Autodesk Inventor part; units mm, degrees
(part 2 of 3)
  spline S34 degree 3 poles (-443.5829, -422.363) (-442.2822, -421.8669) (-439.6808, -420.8747) (-435.8139, -419.2967) (-431.976, -417.6498) (-428.1717, -415.9263) (-424.4077, -414.1171) (-421.6079, -412.712) (-419.7704, -411.7206) (-418.9626, -411.3892) (-418.2875, -411.2153) (-417.7698, -411.1447) (-417.2482, -411.1077) (-416.7264, -411.1464) (-416.21, -411.2266) (-415.7059, -411.3678) (-415.2255, -411.5743) (-414.7643, -411.82) (-414.3345, -412.1194) (-413.8232, -412.5931) (-413.2204, -413.2204) (-412.5931, -413.8232) (-412.1194, -414.3345) (-411.82, -414.7643) (-411.5743, -415.2255) (-411.3678, -415.7059) (-411.2266, -416.21) (-411.1464, -416.7264) (-411.1077, -417.2482) (-411.1447, -417.7698) (-411.2153, -418.2875) (-411.3892, -418.9626) (-411.7206, -419.7704) (-412.712, -421.6079) (-414.1171, -424.4077) (-415.9263, -428.1717) (-417.6498, -431.976) (-419.2967, -435.8139) (-420.8747, -439.6808) (-421.8669, -442.2822) (-422.363, -443.5829) knots 0 0 0 0 0.062504 0.125008 0.187512 0.250016 0.31252 0.375023 0.390648 0.406259 0.414073 0.421883 0.429693 0.437504 0.445316 0.453129 0.460938 0.468749 0.476563 0.484374 0.5 0.515626 0.523437 0.531251 0.539062 0.546871 0.554684 0.562496 0.570307 0.578117 0.585927 0.593741 0.609352 0.624977 0.68748 0.749984 0.812488 0.874992 0.937496 1 1 1 1 projected
  arc A38 (-422.363, -443.5829) -> (-415.0093, -450.4704) centre (0, 0) ccw projected
  spline S35 degree 3 poles (-415.0093, -450.4704) (-413.7438, -449.8903) (-411.2129, -448.73) (-407.4575, -446.9025) (-403.7355, -445.0082) (-400.0521, -443.0396) (-396.4144, -440.988) (-393.7126, -439.4028) (-391.9438, -438.2934) (-391.1594, -437.9098) (-390.4971, -437.6922) (-389.9852, -437.5879) (-389.4671, -437.5168) (-388.9439, -437.5214) (-388.4234, -437.5676) (-387.9111, -437.6755) (-387.4182, -437.8501) (-386.9419, -438.0652) (-386.4935, -438.3358) (-385.9523, -438.775) (-385.3098, -439.3616) (-384.6444, -439.922) (-384.1382, -440.4013) (-383.8114, -440.8106) (-383.5361, -441.2547) (-383.2986, -441.7205) (-383.1247, -442.2144) (-383.0109, -442.7244) (-382.9381, -443.2425) (-382.941, -443.7655) (-382.9776, -444.2867) (-383.1069, -444.9717) (-383.3848, -445.7994) (-384.2539, -447.6979) (-385.4728, -450.5835) (-387.032, -454.4578) (-388.503, -458.3667) (-389.8954, -462.3041) (-391.217, -466.266) (-392.037, -468.9267) (-392.4469, -470.257) knots 0 0 0 0 0.062504 0.125008 0.187512 0.250016 0.31252 0.375023 0.390648 0.406259 0.414073 0.421883 0.429693 0.437504 0.445316 0.453129 0.460938 0.468749 0.476563 0.484374 0.5 0.515626 0.523437 0.531251 0.539062 0.546871 0.554684 0.562496 0.570307 0.578117 0.585927 0.593741 0.609352 0.624977 0.68748 0.749984 0.812488 0.874992 0.937496 1 1 1 1 projected
  arc A39 (-392.4469, -470.257) -> (-384.6585, -476.6488) centre (0, 0) ccw projected
  spline S36 degree 3 poles (-384.6585, -476.6488) (-383.4337, -475.9871) (-380.9841, -474.6639) (-377.3563, -472.5947) (-373.7661, -470.461) (-370.2193, -468.2556) (-366.7237, -465.9706) (-364.1313, -464.2121) (-362.4389, -462.9893) (-361.6812, -462.5553) (-361.0346, -462.2948) (-360.5306, -462.1572) (-360.0182, -462.0524) (-359.4958, -462.0227) (-358.9735, -462.0348) (-358.4552, -462.109) (-357.952, -462.251) (-357.4626, -462.4345) (-356.9975, -462.6752) (-356.4287, -463.0781) (-355.7492, -463.6214) (-355.0485, -464.1371) (-354.5121, -464.5822) (-354.1592, -464.9692) (-353.8554, -465.3944) (-353.588, -465.8437) (-353.3822, -466.3252) (-353.2353, -466.8266) (-353.1288, -467.3389) (-353.0974, -467.8609) (-353.0998, -468.3833) (-353.1841, -469.0753) (-353.4072, -469.9195) (-354.1503, -471.8707) (-355.1779, -474.8299) (-356.4804, -478.7979) (-357.6926, -482.7946) (-358.8244, -486.8147) (-359.8842, -490.8545) (-360.5283, -493.5631) (-360.8504, -494.9174) knots 0 0 0 0 0.062504 0.125008 0.187512 0.250016 0.31252 0.375023 0.390648 0.406259 0.414073 0.421883 0.429693 0.437504 0.445316 0.453129 0.460938 0.468749 0.476563 0.484374 0.5 0.515626 0.523437 0.531251 0.539062 0.546871 0.554684 0.562496 0.570307 0.578117 0.585927 0.593741 0.609352 0.624977 0.68748 0.749984 0.812488 0.874992 0.937496 1 1 1 1 projected
  arc A40 (-360.8504, -494.9174) -> (-352.6606, -500.7861) centre (0, 0) ccw projected
  spline S37 degree 3 poles (-352.6606, -500.7861) (-351.4817, -500.0458) (-349.1239, -498.5651) (-345.6391, -496.2631) (-342.1963, -493.8992) (-338.8013, -491.4666) (-335.4626, -488.9578) (-332.9907, -487.0335) (-331.3819, -485.7026) (-330.6543, -485.22) (-330.0261, -484.9178) (-329.5321, -484.7475) (-329.0277, -484.6094) (-328.5084, -484.5457) (-327.9863, -484.5236) (-327.4643, -484.5637) (-326.9529, -484.6725) (-326.4526, -484.8235) (-325.9727, -485.0333) (-325.3788, -485.3981) (-324.6652, -485.8958) (-323.9323, -486.3646) (-323.368, -486.7737) (-322.9905, -487.1368) (-322.6596, -487.5412) (-322.3633, -487.9721) (-322.1265, -488.439) (-321.9471, -488.9298) (-321.8073, -489.434) (-321.7418, -489.9528) (-321.7101, -490.4743) (-321.7489, -491.1704) (-321.9163, -492.0273) (-322.5302, -494.023) (-323.3621, -497.043) (-324.4023, -501.0877) (-325.3505, -505.1551) (-326.217, -509.2406) (-327.0102, -513.3411) (-327.4758, -516.086) (-327.7086, -517.4585) knots 0 0 0 0 0.062504 0.125008 0.187512 0.250016 0.31252 0.375023 0.390648 0.406259 0.414073 0.421883 0.429693 0.437504 0.445316 0.453129 0.460938 0.468749 0.476563 0.484374 0.5 0.515626 0.523437 0.531251 0.539062 0.546871 0.554684 0.562496 0.570307 0.578117 0.585927 0.593741 0.609352 0.624977 0.68748 0.749984 0.812488 0.874992 0.937496 1 1 1 1 projected
  arc A41 (-327.7086, -517.4585) -> (-319.1526, -522.779) centre (0, 0) ccw projected
  spline S38 degree 3 poles (-319.1526, -522.779) (-318.0246, -521.9632) (-315.7687, -520.3315) (-312.4419, -517.8064) (-309.161, -515.2224) (-305.9324, -512.573) (-302.765, -509.8512) (-300.4243, -507.7693) (-298.9059, -506.3361) (-298.2114, -505.8069) (-297.6043, -505.4643) (-297.1225, -505.2621) (-296.6283, -505.0913) (-296.1142, -504.9937) (-295.5947, -504.9375) (-295.0712, -504.9434) (-294.5538, -505.0185) (-294.0447, -505.1365) (-293.5521, -505.3144) (-292.9356, -505.6397) (-292.191, -506.0896) (-291.429, -506.5095) (-290.8391, -506.8808) (-290.4387, -507.2184) (-290.082, -507.6003) (-289.7582, -508.0108) (-289.4913, -508.4613) (-289.2802, -508.9393) (-289.1077, -509.4333) (-289.0085, -509.9467) (-288.9427, -510.465) (-288.936, -511.1621) (-289.047, -512.0282) (-289.529, -514.0597) (-290.1616, -517.1277) (-290.935, -521.2318) (-291.6152, -525.3525) (-292.2126, -529.4859) (-292.7359, -533.6295) (-293.021, -536.399) (-293.1636, -537.7837) knots 0 0 0 0 0.062504 0.125008 0.187512 0.250016 0.31252 0.375023 0.390648 0.406259 0.414073 0.421883 0.429693 0.437504 0.445316 0.453129 0.460938 0.468749 0.476563 0.484374 0.5 0.515626 0.523437 0.531251 0.539062 0.546871 0.554684 0.562496 0.570307 0.578117 0.585927 0.593741 0.609352 0.624977 0.68748 0.749984 0.812488 0.874992 0.937496 1 1 1 1 projected
  arc A42 (-293.1636, -537.7837) -> (-284.2779, -542.5333) centre (0, 0) ccw projected
  spline S39 degree 3 poles (-284.2779, -542.5333) (-283.2057, -541.6454) (-281.0613, -539.8697) (-277.9068, -537.1325) (-274.802, -534.3394) (-271.7535, -531.4845) (-268.7708, -528.5613) (-266.5713, -526.3309) (-265.15, -524.8014) (-264.4916, -524.2279) (-263.9082, -523.8463) (-263.4407, -523.613) (-262.9586, -523.4103) (-262.4521, -523.2793) (-261.9374, -523.1892) (-261.4146, -523.1608) (-260.8933, -523.202) (-260.3776, -523.2864) (-259.8744, -523.4317) (-259.2379, -523.7159) (-258.4655, -524.1162) (-257.6777, -524.4854) (-257.0648, -524.8173) (-256.6432, -525.128) (-256.2623, -525.4858) (-255.9123, -525.8742) (-255.6166, -526.3063) (-255.3746, -526.7694) (-255.1702, -527.2511) (-255.0376, -527.7569) (-254.9381, -528.2698) (-254.8857, -528.965) (-254.9399, -529.8365) (-255.288, -531.8952) (-255.7186, -534.998) (-256.2219, -539.1438) (-256.6311, -543.3002) (-256.9569, -547.4638) (-257.2081, -551.6328) (-257.3115, -554.415) (-257.3632, -555.8061) knots 0 0 0 0 0.062504 0.125008 0.187512 0.250016 0.31252 0.375023 0.390648 0.406259 0.414073 0.421883 0.429693 0.437504 0.445316 0.453129 0.460938 0.468749 0.476563 0.484374 0.5 0.515626 0.523437 0.531251 0.539062 0.546871 0.554684 0.562496 0.570307 0.578117 0.585927 0.593741 0.609352 0.624977 0.68748 0.749984 0.812488 0.874992 0.937496 1 1 1 1 projected
  arc A43 (-257.3632, -555.8061) -> (-248.1858, -559.9643) centre (0, 0) ccw projected
  spline S40 degree 3 poles (-248.1858, -559.9643) (-247.174, -559.0082) (-245.1504, -557.0961) (-242.1816, -554.1584) (-239.2661, -551.1682) (-236.411, -548.12) (-233.6258, -545.0081) (-231.5769, -542.6385) (-230.2586, -541.0194) (-229.6391, -540.4041) (-229.0819, -539.9851) (-228.6307, -539.7217) (-228.1629, -539.4879) (-227.666, -539.3241) (-227.1583, -539.2006) (-226.6385, -539.138) (-226.1157, -539.145) (-225.5955, -539.1955) (-225.0839, -539.3076) (-224.4302, -539.5496) (-223.6333, -539.8985) (-222.823, -540.2153) (-222.1897, -540.5064) (-221.7487, -540.7889) (-221.3452, -541.121) (-220.9705, -541.4858) (-220.6472, -541.8976) (-220.3755, -542.3439) (-220.14, -542.8111) (-219.9746, -543.3072) (-219.8417, -543.8125) (-219.744, -544.5028) (-219.741, -545.3759) (-219.9538, -547.453) (-220.1805, -550.5773) (-220.4116, -554.7472) (-220.5481, -558.9215) (-220.6009, -563.0974) (-220.5789, -567.2739) (-220.5001, -570.0569) (-220.4607, -571.4485) knots 0 0 0 0 0.062504 0.125008 0.187512 0.250016 0.31252 0.375023 0.390648 0.406259 0.414073 0.421883 0.429693 0.437504 0.445316 0.453129 0.460938 0.468749 0.476563 0.484374 0.5 0.515626 0.523437 0.531251 0.539062 0.546871 0.554684 0.562496 0.570307 0.578117 0.585927 0.593741 0.609352 0.624977 0.68748 0.749984 0.812488 0.874992 0.937496 1 1 1 1 projected
  arc A44 (-220.4607, -571.4485) -> (-211.031, -574.9975) centre (0, 0) ccw projected
  spline S41 degree 3 poles (-211.031, -574.9975) (-210.0839, -573.9773) (-208.1897, -571.9369) (-205.4194, -568.8113) (-202.7057, -565.6369) (-200.056, -562.4085) (-197.4804, -559.121) (-195.5908, -556.6226) (-194.3813, -554.9207) (-193.8033, -554.2662) (-193.2747, -553.8116) (-192.8417, -553.5193) (-192.3902, -553.2554) (-191.9051, -553.0594) (-191.4066, -552.903) (-190.8919, -552.8066) (-190.3698, -552.7793) (-189.8475, -552.7957) (-189.3296, -552.8741) (-188.6615, -553.0728) (-187.8434, -553.3689) (-187.0142, -553.632) (-186.3632, -553.8811) (-185.9046, -554.1341) (-185.4802, -554.4391) (-185.0826, -554.7786) (-184.733, -555.1683) (-184.4327, -555.5959) (-184.1671, -556.0468) (-183.9696, -556.531) (-183.804, -557.0265) (-183.6613, -557.7089) (-183.6013, -558.58) (-183.6777, -560.6665) (-183.6996, -563.799) (-183.6575, -567.975) (-183.5207, -572.1493) (-183.3002, -576.3198) (-183.0051, -580.4859) (-182.7445, -583.2578) (-182.6141, -584.6438) knots 0 0 0 0 0.062504 0.125008 0.187512 0.250016 0.31252 0.375023 0.390648 0.406259 0.414073 0.421883 0.429693 0.437504 0.445316 0.453129 0.460938 0.468749 0.476563 0.484374 0.5 0.515626 0.523437 0.531251 0.539062 0.546871 0.554684 0.562496 0.570307 0.578117 0.585927 0.593741 0.609352 0.624977 0.68748 0.749984 0.812488 0.874992 0.937496 1 1 1 1 projected
  arc A45 (-182.6141, -584.6438) -> (-172.9726, -587.5685) centre (0, 0) ccw projected
  spline S42 degree 3 poles (-172.9726, -587.5685) (-172.0942, -586.4885) (-170.3374, -584.3286) (-167.7776, -581.0285) (-165.2773, -577.6834) (-162.8444, -574.2886) (-160.4893, -570.8398) (-158.7672, -568.223) (-157.6715, -566.4457) (-157.1376, -565.7548) (-156.6399, -565.2666) (-156.2269, -564.9466) (-155.7937, -564.6538) (-155.3224, -564.4264) (-154.8352, -564.2377) (-154.3279, -564.1079) (-153.8087, -564.0466) (-153.2864, -564.0288) (-152.7645, -564.0731) (-152.0848, -564.2277) (-151.2492, -564.4696) (-150.4045, -564.6779) (-149.7386, -564.8839) (-149.2645, -565.1064) (-148.8211, -565.383) (-148.402, -565.6957) (-148.0277, -566.0618) (-147.7001, -566.4688) (-147.4056, -566.9013) (-147.1769, -567.3716) (-146.9792, -567.8552) (-146.7922, -568.5268) (-146.6753, -569.3921) (-146.6151, -571.4792) (-146.4321, -574.6064) (-146.1169, -578.7707) (-145.7074, -582.9271) (-145.2146, -587.0743) (-144.6477, -591.2121) (-144.2063, -593.9611) (-143.9856, -595.3355) knots 0 0 0 0 0.062504 0.125008 0.187512 0.250016 0.31252 0.375023 0.390648 0.406259 0.414073 0.421883 0.429693 0.437504 0.445316 0.453129 0.460938 0.468749 0.476563 0.484374 0.5 0.515626 0.523437 0.531251 0.539062 0.546871 0.554684 0.562496 0.570307 0.578117 0.585927 0.593741 0.609352 0.624977 0.68748 0.749984 0.812488 0.874992 0.937496 1 1 1 1 projected
  arc A46 (-143.9856, -595.3355) -> (-134.1734, -597.6234) centre (0, 0) ccw projected
  spline S43 degree 3 poles (-134.1734, -597.6234) (-133.3675, -596.4883) (-131.7558, -594.2181) (-129.4173, -590.7577) (-127.1411, -587.2562) (-124.9355, -583.7096) (-122.811, -580.114) (-121.2637, -577.3903) (-120.2866, -575.5451) (-119.7991, -574.8207) (-119.3343, -574.3011) (-118.9431, -573.9548) (-118.53, -573.6342) (-118.0746, -573.3765) (-117.6007, -573.1564) (-117.1031, -572.9936) (-116.5889, -572.8985) (-116.069, -572.8465) (-115.5453, -572.8567) (-114.857, -572.9665) (-114.0073, -573.1532) (-113.1508, -573.3059) (-112.4728, -573.4678) (-111.9851, -573.6589) (-111.5246, -573.9058) (-111.086, -574.1905) (-110.6885, -574.5313) (-110.335, -574.916) (-110.0129, -575.3283) (-109.7539, -575.7826) (-109.525, -576.2523) (-109.2945, -576.9102) (-109.1212, -577.766) (-108.9247, -579.8447) (-108.5375, -582.9532) (-107.9507, -587.088) (-107.2701, -591.2087) (-106.5072, -595.3148) (-105.6709, -599.4067) (-105.0506, -602.1209) (-104.7405, -603.478) knots 0 0 0 0 0.062504 0.125008 0.187512 0.250016 0.31252 0.375023 0.390648 0.406259 0.414073 0.421883 0.429693 0.437504 0.445316 0.453129 0.460938 0.468749 0.476563 0.484374 0.5 0.515626 0.523437 0.531251 0.539062 0.546871 0.554684 0.562496 0.570307 0.578117 0.585927 0.593741 0.609352 0.624977 0.68748 0.749984 0.812488 0.874992 0.937496 1 1 1 1 projected
  arc A47 (-104.7405, -603.478) -> (-94.7997, -605.1192) centre (0, 0) ccw projected
  spline S44 degree 3 poles (-94.7997, -605.1192) (-94.0698, -603.9338) (-92.61, -601.5631) (-90.5028, -597.9571) (-88.4605, -594.3142) (-86.4915, -590.631) (-84.6067, -586.9042) (-83.2409, -584.0851) (-82.3866, -582.1799) (-81.9475, -581.4252) (-81.5177, -580.8763) (-81.15, -580.5051) (-80.7587, -580.1582) (-80.3212, -579.8713) (-79.8627, -579.6206) (-79.3768, -579.4257) (-78.87, -579.2971) (-78.3545, -579.2113) (-77.8313, -579.1872) (-77.1372, -579.2517) (-76.2772, -579.3825) (-75.4125, -579.4788) (-74.7254, -579.5961) (-74.2263, -579.7548) (-73.7506, -579.9711) (-73.2943, -580.2265) (-72.8754, -580.5405) (-72.4975, -580.9014) (-72.1491, -581.2917) (-71.8609, -581.7281) (-71.6018, -582.1818) (-71.3287, -582.8232) (-71.0999, -583.6659) (-70.7678, -585.7272) (-70.1781, -588.8038) (-69.3221, -592.8914) (-68.3736, -596.9587) (-67.3437, -601.0061) (-66.2416, -605.0345) (-65.4451, -607.7023) (-65.0469, -609.0362) knots 0 0 0 0 0.062504 0.125008 0.187512 0.250016 0.31252 0.375023 0.390648 0.406259 0.414073 0.421883 0.429693 0.437504 0.445316 0.453129 0.460938 0.468749 0.476563 0.484374 0.5 0.515626 0.523437 0.531251 0.539062 0.546871 0.554684 0.562496 0.570307 0.578117 0.585927 0.593741 0.609352 0.624977 0.68748 0.749984 0.812488 0.874992 0.937496 1 1 1 1 projected
  arc A48 (-65.0469, -609.0362) -> (-55.02, -610.0238) centre (0, 0) ccw projected
  spline S45 degree 3 poles (-55.02, -610.0238) (-54.3692, -608.7932) (-53.0676, -606.332) (-51.2007, -602.596) (-49.4011, -598.8274) (-47.6772, -595.0232) (-46.0402, -591.1811) (-44.8617, -588.2787) (-44.1338, -586.3218) (-43.745, -585.54) (-43.3521, -584.9641) (-43.0094, -584.5697) (-42.6417, -584.1979) (-42.2238, -583.883) (-41.7827, -583.6029) (-41.3106, -583.3766) (-40.8133, -583.2151) (-40.3045, -583.0958) (-39.784, -583.0375) (-39.0872, -583.0565) (-38.2204, -583.1308) (-37.3513, -583.1703) (-36.658, -583.2424) (-36.1496, -583.3681) (-35.6608, -583.5529) (-35.1888, -583.7778) (-34.7502, -584.0638) (-34.3495, -584.3992) (-33.9763, -584.7659) (-33.6602, -585.1825) (-33.3719, -585.6183) (-33.0576, -586.2405) (-32.7741, -587.0663) (-32.3079, -589.1016) (-31.5183, -592.133) (-30.3968, -596.1558) (-29.1842, -600.1524) (-27.8919, -604.1238) (-26.5286, -608.0715) (-25.5594, -610.6815) (-25.0748, -611.9865) knots 0 0 0 0 0.062504 0.125008 0.187512 0.250016 0.31252 0.375023 0.390648 0.406259 0.414073 0.421883 0.429693 0.437504 0.445316 0.453129 0.460938 0.468749 0.476563 0.484374 0.5 0.515626 0.523437 0.531251 0.539062 0.546871 0.554684 0.562496 0.570307 0.578117 0.585927 0.593741 0.609352 0.624977 0.68748 0.749984 0.812488 0.874992 0.937496 1 1 1 1 projected
  arc A49 (-25.0748, -611.9865) -> (-15.0048, -612.3162) centre (0, 0) ccw projected
  spline S46 degree 3 poles (-15.0048, -612.3162) (-14.4358, -611.0457) (-13.298, -608.5046) (-11.6794, -604.6545) (-10.1301, -600.7762) (-8.6588, -596.8674) (-7.2766, -592.9265) (-6.2904, -589.9533) (-5.6921, -587.9529) (-5.3552, -587.1474) (-5.0008, -586.547) (-4.6846, -586.131) (-4.342, -585.736) (-3.9456, -585.3945) (-3.5238, -585.0861) (-3.0675, -584.8294) (-2.5818, -584.6357) (-2.0819, -584.4834) (-1.5663, -584.3912) (-0.8698, -584.3646) (0, -584.382) (0.8698, -584.3646) (1.5663, -584.3912) (2.0819, -584.4834) (2.5818, -584.6357) (3.0675, -584.8294) (3.5238, -585.0861) (3.9456, -585.3945) (4.342, -585.736) (4.6846, -586.131) (5.0008, -586.547) (5.3552, -587.1474) (5.6921, -587.9529) (6.2904, -589.9533) (7.2766, -592.9265) (8.6588, -596.8674) (10.1301, -600.7762) (11.6794, -604.6545) (13.298, -608.5046) (14.4358, -611.0457) (15.0048, -612.3162) knots 0 0 0 0 0.062504 0.125008 0.187512 0.250016 0.31252 0.375023 0.390648 0.406259 0.414073 0.421883 0.429693 0.437504 0.445316 0.453129 0.460938 0.468749 0.476563 0.484374 0.5 0.515626 0.523437 0.531251 0.539062 0.546871 0.554684 0.562496 0.570307 0.578117 0.585927 0.593741 0.609352 0.624977 0.68748 0.749984 0.812488 0.874992 0.937496 1 1 1 1 projected
  arc A50 (15.0048, -612.3162) -> (25.0748, -611.9865) centre (0, 0) ccw projected
  spline S47 degree 3 poles (25.0748, -611.9865) (25.5594, -610.6815) (26.5286, -608.0715) (27.8919, -604.1238) (29.1842, -600.1524) (30.3968, -596.1558) (31.5183, -592.133) (32.3079, -589.1016) (32.7741, -587.0663) (33.0576, -586.2405) (33.3719, -585.6183) (33.6602, -585.1825) (33.9763, -584.7659) (34.3495, -584.3992) (34.7502, -584.0638) (35.1888, -583.7778) (35.6608, -583.5529) (36.1496, -583.3681) (36.658, -583.2424) (37.3513, -583.1703) (38.2204, -583.1308) (39.0872, -583.0565) (39.784, -583.0375) (40.3045, -583.0958) (40.8133, -583.2151) (41.3106, -583.3766) (41.7827, -583.6029) (42.2238, -583.883) (42.6417, -584.1979) (43.0094, -584.5697) (43.3521, -584.9641) (43.745, -585.54) (44.1338, -586.3218) (44.8617, -588.2787) (46.0402, -591.1811) (47.6772, -595.0232) (49.4011, -598.8274) (51.2007, -602.596) (53.0676, -606.332) (54.3692, -608.7932) (55.02, -610.0238) knots 0 0 0 0 0.062504 0.125008 0.187512 0.250016 0.31252 0.375023 0.390648 0.406259 0.414073 0.421883 0.429693 0.437504 0.445316 0.453129 0.460938 0.468749 0.476563 0.484374 0.5 0.515626 0.523437 0.531251 0.539062 0.546871 0.554684 0.562496 0.570307 0.578117 0.585927 0.593741 0.609352 0.624977 0.68748 0.749984 0.812488 0.874992 0.937496 1 1 1 1 projected
  arc A51 (55.02, -610.0238) -> (65.0469, -609.0362) centre (0, 0) ccw projected
  spline S48 degree 3 poles (65.0469, -609.0362) (65.4451, -607.7023) (66.2416, -605.0345) (67.3437, -601.0061) (68.3736, -596.9587) (69.3221, -592.8914) (70.1781, -588.8038) (70.7678, -585.7272) (71.0999, -583.6659) (71.3287, -582.8232) (71.6018, -582.1818) (71.8609, -581.7281) (72.1491, -581.2917) (72.4975, -580.9014) (72.8754, -580.5405) (73.2943, -580.2265) (73.7506, -579.9711) (74.2263, -579.7548) (74.7254, -579.5961) (75.4125, -579.4788) (76.2772, -579.3825) (77.1372, -579.2517) (77.8313, -579.1872) (78.3545, -579.2113) (78.87, -579.2971) (79.3768, -579.4257) (79.8627, -579.6206) (80.3212, -579.8713) (80.7587, -580.1582) (81.15, -580.5051) (81.5177, -580.8763) (81.9475, -581.4252) (82.3866, -582.1799) (83.2409, -584.0851) (84.6067, -586.9042) (86.4915, -590.631) (88.4605, -594.3142) (90.5028, -597.9571) (92.61, -601.5631) (94.0698, -603.9338) (94.7997, -605.1192) knots 0 0 0 0 0.062504 0.125008 0.187512 0.250016 0.31252 0.375023 0.390648 0.406259 0.414073 0.421883 0.429693 0.437504 0.445316 0.453129 0.460938 0.468749 0.476563 0.484374 0.5 0.515626 0.523437 0.531251 0.539062 0.546871 0.554684 0.562496 0.570307 0.578117 0.585927 0.593741 0.609352 0.624977 0.68748 0.749984 0.812488 0.874992 0.937496 1 1 1 1 projected
  arc A52 (94.7997, -605.1192) -> (104.7405, -603.478) centre (0, 0) ccw projected
  spline S49 degree 3 poles (104.7405, -603.478) (105.0506, -602.1209) (105.6709, -599.4067) (106.5072, -595.3148) (107.2701, -591.2087) (107.9507, -587.088) (108.5375, -582.9532) (108.9247, -579.8447) (109.1212, -577.766) (109.2945, -576.9102) (109.525, -576.2523) (109.7539, -575.7826) (110.0129, -575.3283) (110.335, -574.916) (110.6885, -574.5313) (111.086, -574.1905) (111.5246, -573.9058) (111.9851, -573.6589) (112.4728, -573.4678) (113.1508, -573.3059) (114.0073, -573.1532) (114.857, -572.9665) (115.5453, -572.8567) (116.069, -572.8465) (116.5889, -572.8985) (117.1031, -572.9936) (117.6007, -573.1564) (118.0746, -573.3765) (118.53, -573.6342) (118.9431, -573.9548) (119.3343, -574.3011) (119.7991, -574.8207) (120.2866, -575.5451) (121.2637, -577.3903) (122.811, -580.114) (124.9355, -583.7096) (127.1411, -587.2562) (129.4173, -590.7577) (131.7558, -594.2181) (133.3675, -596.4883) (134.1734, -597.6234) knots 0 0 0 0 0.062504 0.125008 0.187512 0.250016 0.31252 0.375023 0.390648 0.406259 0.414073 0.421883 0.429693 0.437504 0.445316 0.453129 0.460938 0.468749 0.476563 0.484374 0.5 0.515626 0.523437 0.531251 0.539062 0.546871 0.554684 0.562496 0.570307 0.578117 0.585927 0.593741 0.609352 0.624977 0.68748 0.749984 0.812488 0.874992 0.937496 1 1 1 1 projected
  arc A53 (134.1734, -597.6234) -> (143.9856, -595.3355) centre (0, 0) ccw projected
  spline S50 degree 3 poles (143.9856, -595.3355) (144.2063, -593.9611) (144.6477, -591.2121) (145.2146, -587.0743) (145.7074, -582.9271) (146.1169, -578.7707) (146.4321, -574.6064) (146.6151, -571.4792) (146.6753, -569.3921) (146.7922, -568.5268) (146.9792, -567.8552) (147.1769, -567.3716) (147.4056, -566.9013) (147.7001, -566.4688) (148.0277, -566.0618) (148.402, -565.6957) (148.8211, -565.383) (149.2645, -565.1064) (149.7386, -564.8839) (150.4045, -564.6779) (151.2492, -564.4696) (152.0848, -564.2277) (152.7645, -564.0731) (153.2864, -564.0288) (153.8087, -564.0466) (154.3279, -564.1079) (154.8352, -564.2377) (155.3224, -564.4264) (155.7937, -564.6538) (156.2269, -564.9466) (156.6399, -565.2666) (157.1376, -565.7548) (157.6715, -566.4457) (158.7672, -568.223) (160.4893, -570.8398) (162.8444, -574.2886) (165.2773, -577.6834) (167.7776, -581.0285) (170.3374, -584.3286) (172.0942, -586.4885) (172.9726, -587.5685) knots 0 0 0 0 0.062504 0.125008 0.187512 0.250016 0.31252 0.375023 0.390648 0.406259 0.414073 0.421883 0.429693 0.437504 0.445316 0.453129 0.460938 0.468749 0.476563 0.484374 0.5 0.515626 0.523437 0.531251 0.539062 0.546871 0.554684 0.562496 0.570307 0.578117 0.585927 0.593741 0.609352 0.624977 0.68748 0.749984 0.812488 0.874992 0.937496 1 1 1 1 projected
  arc A54 (172.9726, -587.5685) -> (182.6141, -584.6438) centre (0, 0) ccw projected
  spline S51 degree 3 poles (182.6141, -584.6438) (182.7445, -583.2578) (183.0051, -580.4859) (183.3002, -576.3198) (183.5207, -572.1493) (183.6575, -567.975) (183.6996, -563.799) (183.6777, -560.6665) (183.6013, -558.58) (183.6613, -557.7089) (183.804, -557.0265) (183.9696, -556.531) (184.1671, -556.0468) (184.4327, -555.5959) (184.733, -555.1683) (185.0826, -554.7786) (185.4802, -554.4391) (185.9046, -554.1341) (186.3632, -553.8811) (187.0142, -553.632) (187.8434, -553.3689) (188.6615, -553.0728) (189.3296, -552.8741) (189.8475, -552.7957) (190.3698, -552.7793) (190.8919, -552.8066) (191.4066, -552.903) (191.9051, -553.0594) (192.3902, -553.2554) (192.8417, -553.5193) (193.2747, -553.8116) (193.8033, -554.2662) (194.3813, -554.9207) (195.5908, -556.6226) (197.4804, -559.121) (200.056, -562.4085) (202.7057, -565.6369) (205.4194, -568.8113) (208.1897, -571.9369) (210.0839, -573.9773) (211.031, -574.9975) knots 0 0 0 0 0.062504 0.125008 0.187512 0.250016 0.31252 0.375023 0.390648 0.406259 0.414073 0.421883 0.429693 0.437504 0.445316 0.453129 0.460938 0.468749 0.476563 0.484374 0.5 0.515626 0.523437 0.531251 0.539062 0.546871 0.554684 0.562496 0.570307 0.578117 0.585927 0.593741 0.609352 0.624977 0.68748 0.749984 0.812488 0.874992 0.937496 1 1 1 1 projected
  arc A55 (211.031, -574.9975) -> (220.4607, -571.4485) centre (0, 0) ccw projected
  spline S52 degree 3 poles (220.4607, -571.4485) (220.5001, -570.0569) (220.5789, -567.2739) (220.6009, -563.0974) (220.5481, -558.9215) (220.4116, -554.7472) (220.1805, -550.5773) (219.9538, -547.453) (219.741, -545.3759) (219.744, -544.5028) (219.8417, -543.8125) (219.9746, -543.3072) (220.14, -542.8111) (220.3755, -542.3439) (220.6472, -541.8976) (220.9705, -541.4858) (221.3452, -541.121) (221.7487, -540.7889) (222.1897, -540.5064) (222.823, -540.2153) (223.6333, -539.8985) (224.4302, -539.5496) (225.0839, -539.3076) (225.5955, -539.1955) (226.1157, -539.145) (226.6385, -539.138) (227.1583, -539.2006) (227.666, -539.3241) (228.1629, -539.4879) (228.6307, -539.7217) (229.0819, -539.9851) (229.6391, -540.4041) (230.2586, -541.0194) (231.5769, -542.6385) (233.6258, -545.0081) (236.411, -548.12) (239.2661, -551.1682) (242.1816, -554.1584) (245.1504, -557.0961) (247.174, -559.0082) (248.1858, -559.9643) knots 0 0 0 0 0.062504 0.125008 0.187512 0.250016 0.31252 0.375023 0.390648 0.406259 0.414073 0.421883 0.429693 0.437504 0.445316 0.453129 0.460938 0.468749 0.476563 0.484374 0.5 0.515626 0.523437 0.531251 0.539062 0.546871 0.554684 0.562496 0.570307 0.578117 0.585927 0.593741 0.609352 0.624977 0.68748 0.749984 0.812488 0.874992 0.937496 1 1 1 1 projected
  arc A56 (248.1858, -559.9643) -> (257.3632, -555.8061) centre (0, 0) ccw projected
  spline S53 degree 3 poles (257.3632, -555.8061) (257.3115, -554.415) (257.2081, -551.6328) (256.9569, -547.4638) (256.6311, -543.3002) (256.2219, -539.1438) (255.7186, -534.998) (255.288, -531.8952) (254.9399, -529.8365) (254.8857, -528.965) (254.9381, -528.2698) (255.0376, -527.7569) (255.1702, -527.2511) (255.3746, -526.7694) (255.6166, -526.3063) (255.9123, -525.8742) (256.2623, -525.4858) (256.6432, -525.128) (257.0648, -524.8173) (257.6777, -524.4854) (258.4655, -524.1162) (259.2379, -523.7159) (259.8744, -523.4317) (260.3776, -523.2864) (260.8933, -523.202) (261.4146, -523.1608) (261.9374, -523.1892) (262.4521, -523.2793) (262.9586, -523.4103) (263.4407, -523.613) (263.9082, -523.8463) (264.4916, -524.2279) (265.15, -524.8014) (266.5713, -526.3309) (268.7708, -528.5613) (271.7535, -531.4845) (274.802, -534.3394) (277.9068, -537.1325) (281.0613, -539.8697) (283.2057, -541.6454) (284.2779, -542.5333) knots 0 0 0 0 0.062504 0.125008 0.187512 0.250016 0.31252 0.375023 0.390648 0.406259 0.414073 0.421883 0.429693 0.437504 0.445316 0.453129 0.460938 0.468749 0.476563 0.484374 0.5 0.515626 0.523437 0.531251 0.539062 0.546871 0.554684 0.562496 0.570307 0.578117 0.585927 0.593741 0.609352 0.624977 0.68748 0.749984 0.812488 0.874992 0.937496 1 1 1 1 projected
  arc A57 (284.2779, -542.5333) -> (293.1636, -537.7837) centre (0, 0) ccw projected
  spline S54 degree 3 poles (293.1636, -537.7837) (293.021, -536.399) (292.7359, -533.6295) (292.2126, -529.4859) (291.6152, -525.3525) (290.935, -521.2318) (290.1616, -517.1277) (289.529, -514.0597) (289.047, -512.0282) (288.936, -511.1621) (288.9427, -510.465) (289.0085, -509.9467) (289.1077, -509.4333) (289.2802, -508.9393) (289.4913, -508.4613) (289.7582, -508.0108) (290.082, -507.6003) (290.4387, -507.2184) (290.8391, -506.8808) (291.429, -506.5095) (292.191, -506.0896) (292.9356, -505.6397) (293.5521, -505.3144) (294.0447, -505.1365) (294.5538, -505.0185) (295.0712, -504.9434) (295.5947, -504.9375) (296.1142, -504.9937) (296.6283, -505.0913) (297.1225, -505.2621) (297.6043, -505.4643) (298.2114, -505.8069) (298.9059, -506.3361) (300.4243, -507.7693) (302.765, -509.8512) (305.9324, -512.573) (309.161, -515.2224) (312.4419, -517.8064) (315.7687, -520.3315) (318.0246, -521.9632) (319.1526, -522.779) knots 0 0 0 0 0.062504 0.125008 0.187512 0.250016 0.31252 0.375023 0.390648 0.406259 0.414073 0.421883 0.429693 0.437504 0.445316 0.453129 0.460938 0.468749 0.476563 0.484374 0.5 0.515626 0.523437 0.531251 0.539062 0.546871 0.554684 0.562496 0.570307 0.578117 0.585927 0.593741 0.609352 0.624977 0.68748 0.749984 0.812488 0.874992 0.937496 1 1 1 1 projected
  arc A58 (319.1526, -522.779) -> (327.7086, -517.4585) centre (0, 0) ccw projected
  spline S55 degree 3 poles (327.7086, -517.4585) (327.4758, -516.086) (327.0102, -513.3411) (326.217, -509.2406) (325.3505, -505.1551) (324.4023, -501.0877) (323.3621, -497.043) (322.5302, -494.023) (321.9163, -492.0273) (321.7489, -491.1704) (321.7101, -490.4743) (321.7418, -489.9528) (321.8073, -489.434) (321.9471, -488.9298) (322.1265, -488.439) (322.3633, -487.9721) (322.6596, -487.5412) (322.9905, -487.1368) (323.368, -486.7737) (323.9323, -486.3646) (324.6652, -485.8958) (325.3788, -485.3981) (325.9727, -485.0333) (326.4526, -484.8235) (326.9529, -484.6725) (327.4643, -484.5637) (327.9863, -484.5236) (328.5084, -484.5457) (329.0277, -484.6094) (329.5321, -484.7475) (330.0261, -484.9178) (330.6543, -485.22) (331.3819, -485.7026) (332.9907, -487.0335) (335.4626, -488.9578) (338.8013, -491.4666) (342.1963, -493.8992) (345.6391, -496.2631) (349.1239, -498.5651) (351.4817, -500.0458) (352.6606, -500.7861) knots 0 0 0 0 0.062504 0.125008 0.187512 0.250016 0.31252 0.375023 0.390648 0.406259 0.414073 0.421883 0.429693 0.437504 0.445316 0.453129 0.460938 0.468749 0.476563 0.484374 0.5 0.515626 0.523437 0.531251 0.539062 0.546871 0.554684 0.562496 0.570307 0.578117 0.585927 0.593741 0.609352 0.624977 0.68748 0.749984 0.812488 0.874992 0.937496 1 1 1 1 projected
  arc A59 (352.6606, -500.7861) -> (360.8504, -494.9174) centre (0, 0) ccw projected
  spline S56 degree 3 poles (360.8504, -494.9174) (360.5283, -493.5631) (359.8842, -490.8545) (358.8244, -486.8147) (357.6926, -482.7946) (356.4804, -478.7979) (355.1779, -474.8299) (354.1503, -471.8707) (353.4072, -469.9195) (353.1841, -469.0753) (353.0998, -468.3833) (353.0974, -467.8609) (353.1288, -467.3389) (353.2353, -466.8266) (353.3822, -466.3252) (353.588, -465.8437) (353.8554, -465.3944) (354.1592, -464.9692) (354.5121, -464.5822) (355.0485, -464.1371) (355.7492, -463.6214) (356.4287, -463.0781) (356.9975, -462.6752) (357.4626, -462.4345) (357.952, -462.251) (358.4552, -462.109) (358.9735, -462.0348) (359.4958, -462.0227) (360.0182, -462.0524) (360.5306, -462.1572) (361.0346, -462.2948) (361.6812, -462.5553) (362.4389, -462.9893) (364.1313, -464.2121) (366.7237, -465.9706) (370.2193, -468.2556) (373.7661, -470.461) (377.3563, -472.5947) (380.9841, -474.6639) (383.4337, -475.9871) (384.6585, -476.6488) knots 0 0 0 0 0.062504 0.125008 0.187512 0.250016 0.31252 0.375023 0.390648 0.406259 0.414073 0.421883 0.429693 0.437504 0.445316 0.453129 0.460938 0.468749 0.476563 0.484374 0.5 0.515626 0.523437 0.531251 0.539062 0.546871 0.554684 0.562496 0.570307 0.578117 0.585927 0.593741 0.609352 0.624977 0.68748 0.749984 0.812488 0.874992 0.937496 1 1 1 1 projected
  arc A60 (384.6585, -476.6488) -> (392.4469, -470.257) centre (0, 0) ccw projected
  spline S57 degree 3 poles (392.4469, -470.257) (392.037, -468.9267) (391.217, -466.266) (389.8954, -462.3041) (388.503, -458.3667) (387.032, -454.4578) (385.4728, -450.5835) (384.2539, -447.6979) (383.3848, -445.7994) (383.1069, -444.9717) (382.9776, -444.2867) (382.941, -443.7655) (382.9381, -443.2425) (383.0109, -442.7244) (383.1247, -442.2144) (383.2986, -441.7205) (383.5361, -441.2547) (383.8114, -440.8106) (384.1382, -440.4013) (384.6444, -439.922) (385.3098, -439.3616) (385.9523, -438.775) (386.4935, -438.3358) (386.9419, -438.0652) (387.4182, -437.8501) (387.9111, -437.6755) (388.4234, -437.5676) (388.9439, -437.5214) (389.4671, -437.5168) (389.9852, -437.5879) (390.4971, -437.6922) (391.1594, -437.9098) (391.9438, -438.2934) (393.7126, -439.4028) (396.4144, -440.988) (400.0521, -443.0396) (403.7355, -445.0082) (407.4575, -446.9025) (411.2129, -448.73) (413.7438, -449.8903) (415.0093, -450.4704) knots 0 0 0 0 0.062504 0.125008 0.187512 0.250016 0.31252 0.375023 0.390648 0.406259 0.414073 0.421883 0.429693 0.437504 0.445316 0.453129 0.460938 0.468749 0.476563 0.484374 0.5 0.515626 0.523437 0.531251 0.539062 0.546871 0.554684 0.562496 0.570307 0.578117 0.585927 0.593741 0.609352 0.624977 0.68748 0.749984 0.812488 0.874992 0.937496 1 1 1 1 projected
  arc A61 (415.0093, -450.4704) -> (422.363, -443.5829) centre (0, 0) ccw projected
  spline S58 degree 3 poles (422.363, -443.5829) (421.8669, -442.2822) (420.8747, -439.6808) (419.2967, -435.8139) (417.6498, -431.976) (415.9263, -428.1717) (414.1171, -424.4077) (412.712, -421.6079) (411.7206, -419.7704) (411.3892, -418.9626) (411.2153, -418.2875) (411.1447, -417.7698) (411.1077, -417.2482) (411.1464, -416.7264) (411.2266, -416.21) (411.3678, -415.7059) (411.5743, -415.2255) (411.82, -414.7643) (412.1194, -414.3345) (412.5931, -413.8232) (413.2204, -413.2204) (413.8232, -412.5931) (414.3345, -412.1194) (414.7643, -411.82) (415.2255, -411.5743) (415.7059, -411.3678) (416.21, -411.2266) (416.7264, -411.1464) (417.2482, -411.1077) (417.7698, -411.1447) (418.2875, -411.2153) (418.9626, -411.3892) (419.7704, -411.7206) (421.6079, -412.712) (424.4077, -414.1171) (428.1717, -415.9263) (431.976, -417.6498) (435.8139, -419.2967) (439.6808, -420.8747) (442.2822, -421.8669) (443.5829, -422.363) knots 0 0 0 0 0.062504 0.125008 0.187512 0.250016 0.31252 0.375023 0.390648 0.406259 0.414073 0.421883 0.429693 0.437504 0.445316 0.453129 0.460938 0.468749 0.476563 0.484374 0.5 0.515626 0.523437 0.531251 0.539062 0.546871 0.554684 0.562496 0.570307 0.578117 0.585927 0.593741 0.609352 0.624977 0.68748 0.749984 0.812488 0.874992 0.937496 1 1 1 1 projected
  arc A62 (443.5829, -422.363) -> (450.4704, -415.0093) centre (0, 0) ccw projected
  spline S59 degree 3 poles (450.4704, -415.0093) (449.8903, -413.7438) (448.73, -411.2129) (446.9025, -407.4575) (445.0082, -403.7355) (443.0396, -400.0521) (440.988, -396.4144) (439.4028, -393.7126) (438.2934, -391.9438) (437.9098, -391.1594) (437.6922, -390.4971) (437.5879, -389.9852) (437.5168, -389.4671) (437.5214, -388.9439) (437.5676, -388.4234) (437.6755, -387.9111) (437.8501, -387.4182) (438.0652, -386.9419) (438.3358, -386.4935) (438.775, -385.9523) (439.3616, -385.3098) (439.922, -384.6444) (440.4013, -384.1382) (440.8106, -383.8114) (441.2547, -383.5361) (441.7205, -383.2986) (442.2144, -383.1247) (442.7244, -383.0109) (443.2425, -382.9381) (443.7655, -382.941) (444.2867, -382.9776) (444.9717, -383.1069) (445.7994, -383.3848) (447.6979, -384.2539) (450.5835, -385.4728) (454.4578, -387.032) (458.3667, -388.503) (462.3041, -389.8954) (466.266, -391.217) (468.9267, -392.037) (470.257, -392.4469) knots 0 0 0 0 0.062504 0.125008 0.187512 0.250016 0.31252 0.375023 0.390648 0.406259 0.414073 0.421883 0.429693 0.437504 0.445316 0.453129 0.460938 0.468749 0.476563 0.484374 0.5 0.515626 0.523437 0.531251 0.539062 0.546871 0.554684 0.562496 0.570307 0.578117 0.585927 0.593741 0.609352 0.624977 0.68748 0.749984 0.812488 0.874992 0.937496 1 1 1 1 projected
  arc A63 (470.257, -392.4469) -> (476.6488, -384.6585) centre (0, 0) ccw projected
  spline S60 degree 3 poles (476.6488, -384.6585) (475.9871, -383.4337) (474.6639, -380.9841) (472.5947, -377.3563) (470.461, -373.7661) (468.2556, -370.2193) (465.9706, -366.7237) (464.2121, -364.1313) (462.9893, -362.4389) (462.5553, -361.6812) (462.2948, -361.0346) (462.1572, -360.5306) (462.0524, -360.0182) (462.0227, -359.4958) (462.0348, -358.9735) (462.109, -358.4552) (462.251, -357.952) (462.4345, -357.4626) (462.6752, -356.9975) (463.0781, -356.4287) (463.6214, -355.7492) (464.1371, -355.0485) (464.5822, -354.5121) (464.9692, -354.1592) (465.3944, -353.8554) (465.8437, -353.588) (466.3252, -353.3822) (466.8266, -353.2353) (467.3389, -353.1288) (467.8609, -353.0974) (468.3833, -353.0998) (469.0753, -353.1841) (469.9195, -353.4072) (471.8707, -354.1503) (474.8299, -355.1779) (478.7979, -356.4804) (482.7946, -357.6926) (486.8147, -358.8244) (490.8545, -359.8842) (493.5631, -360.5283) (494.9174, -360.8504) knots 0 0 0 0 0.062504 0.125008 0.187512 0.250016 0.31252 0.375023 0.390648 0.406259 0.414073 0.421883 0.429693 0.437504 0.445316 0.453129 0.460938 0.468749 0.476563 0.484374 0.5 0.515626 0.523437 0.531251 0.539062 0.546871 0.554684 0.562496 0.570307 0.578117 0.585927 0.593741 0.609352 0.624977 0.68748 0.749984 0.812488 0.874992 0.937496 1 1 1 1 projected
  arc A64 (494.9174, -360.8504) -> (500.7861, -352.6606) centre (0, 0) ccw projected
  spline S61 degree 3 poles (500.7861, -352.6606) (500.0458, -351.4817) (498.5651, -349.1239) (496.2631, -345.6391) (493.8992, -342.1963) (491.4666, -338.8013) (488.9578, -335.4626) (487.0335, -332.9907) (485.7026, -331.3819) (485.22, -330.6543) (484.9178, -330.0261) (484.7475, -329.5321) (484.6094, -329.0277) (484.5457, -328.5084) (484.5236, -327.9863) (484.5637, -327.4643) (484.6725, -326.9529) (484.8235, -326.4526) (485.0333, -325.9727) (485.3981, -325.3788) (485.8958, -324.6652) (486.3646, -323.9323) (486.7737, -323.368) (487.1368, -322.9905) (487.5412, -322.6596) (487.9721, -322.3633) (488.439, -322.1265) (488.9298, -321.9471) (489.434, -321.8073) (489.9528, -321.7418) (490.4743, -321.7101) (491.1704, -321.7489) (492.0273, -321.9163) (494.023, -322.5302) (497.043, -323.3621) (501.0877, -324.4023) (505.1551, -325.3505) (509.2406, -326.217) (513.3411, -327.0102) (516.086, -327.4758) (517.4585, -327.7086) knots 0 0 0 0 0.062504 0.125008 0.187512 0.250016 0.31252 0.375023 0.390648 0.406259 0.414073 0.421883 0.429693 0.437504 0.445316 0.453129 0.460938 0.468749 0.476563 0.484374 0.5 0.515626 0.523437 0.531251 0.539062 0.546871 0.554684 0.562496 0.570307 0.578117 0.585927 0.593741 0.609352 0.624977 0.68748 0.749984 0.812488 0.874992 0.937496 1 1 1 1 projected
  arc A65 (517.4585, -327.7086) -> (522.779, -319.1526) centre (0, 0) ccw projected
  spline S62 degree 3 poles (522.779, -319.1526) (521.9632, -318.0246) (520.3315, -315.7687) (517.8064, -312.4419) (515.2224, -309.161) (512.573, -305.9324) (509.8512, -302.765) (507.7693, -300.4243) (506.3361, -298.9059) (505.8069, -298.2114) (505.4643, -297.6043) (505.2621, -297.1225) (505.0913, -296.6283) (504.9937, -296.1142) (504.9375, -295.5947) (504.9434, -295.0712) (505.0185, -294.5538) (505.1365, -294.0447) (505.3144, -293.5521) (505.6397, -292.9356) (506.0896, -292.191) (506.5095, -291.429) (506.8808, -290.8391) (507.2184, -290.4387) (507.6003, -290.082) (508.0108, -289.7582) (508.4613, -289.4913) (508.9393, -289.2802) (509.4333, -289.1077) (509.9467, -289.0085) (510.465, -288.9427) (511.1621, -288.936) (512.0282, -289.047) (514.0597, -289.529) (517.1277, -290.1616) (521.2318, -290.935) (525.3525, -291.6152) (529.4859, -292.2126) (533.6295, -292.7359) (536.399, -293.021) (537.7837, -293.1636) knots 0 0 0 0 0.062504 0.125008 0.187512 0.250016 0.31252 0.375023 0.390648 0.406259 0.414073 0.421883 0.429693 0.437504 0.445316 0.453129 0.460938 0.468749 0.476563 0.484374 0.5 0.515626 0.523437 0.531251 0.539062 0.546871 0.554684 0.562496 0.570307 0.578117 0.585927 0.593741 0.609352 0.624977 0.68748 0.749984 0.812488 0.874992 0.937496 1 1 1 1 projected
  arc A66 (537.7837, -293.1636) -> (542.5333, -284.2779) centre (0, 0) ccw projected
  spline S63 degree 3 poles (542.5333, -284.2779) (541.6454, -283.2057) (539.8697, -281.0613) (537.1325, -277.9068) (534.3394, -274.802) (531.4845, -271.7535) (528.5613, -268.7708) (526.3309, -266.5713) (524.8014, -265.15) (524.2279, -264.4916) (523.8463, -263.9082) (523.613, -263.4407) (523.4103, -262.9586) (523.2793, -262.4521) (523.1892, -261.9374) (523.1608, -261.4146) (523.202, -260.8933) (523.2864, -260.3776) (523.4317, -259.8744) (523.7159, -259.2379) (524.1162, -258.4655) (524.4854, -257.6777) (524.8173, -257.0648) (525.128, -256.6432) (525.4858, -256.2623) (525.8742, -255.9123) (526.3063, -255.6166) (526.7694, -255.3746) (527.2511, -255.1702) (527.7569, -255.0376) (528.2698, -254.9381) (528.965, -254.8857) (529.8365, -254.9399) (531.8952, -255.288) (534.998, -255.7186) (539.1438, -256.2219) (543.3002, -256.6311) (547.4638, -256.9569) (551.6328, -257.2081) (554.415, -257.3115) (555.8061, -257.3632) knots 0 0 0 0 0.062504 0.125008 0.187512 0.250016 0.31252 0.375023 0.390648 0.406259 0.414073 0.421883 0.429693 0.437504 0.445316 0.453129 0.460938 0.468749 0.476563 0.484374 0.5 0.515626 0.523437 0.531251 0.539062 0.546871 0.554684 0.562496 0.570307 0.578117 0.585927 0.593741 0.609352 0.624977 0.68748 0.749984 0.812488 0.874992 0.937496 1 1 1 1 projected
  arc A67 (555.8061, -257.3632) -> (559.9643, -248.1858) centre (0, 0) ccw projected
  spline S64 degree 3 poles (559.9643, -248.1858) (559.0082, -247.174) (557.0961, -245.1504) (554.1584, -242.1816) (551.1682, -239.2661) (548.12, -236.411) (545.0081, -233.6258) (542.6385, -231.5769) (541.0194, -230.2586) (540.4041, -229.6391) (539.9851, -229.0819) (539.7217, -228.6307) (539.4879, -228.1629) (539.3241, -227.666) (539.2006, -227.1583) (539.138, -226.6385) (539.145, -226.1157) (539.1955, -225.5955) (539.3076, -225.0839) (539.5496, -224.4302) (539.8985, -223.6333) (540.2153, -222.823) (540.5064, -222.1897) (540.7889, -221.7487) (541.121, -221.3452) (541.4858, -220.9705) (541.8976, -220.6472) (542.3439, -220.3755) (542.8111, -220.14) (543.3072, -219.9746) (543.8125, -219.8417) (544.5028, -219.744) (545.3759, -219.741) (547.453, -219.9538) (550.5773, -220.1805) (554.7472, -220.4116) (558.9215, -220.5481) (563.0974, -220.6009) (567.2739, -220.5789) (570.0569, -220.5001) (571.4485, -220.4607) knots 0 0 0 0 0.062504 0.125008 0.187512 0.250016 0.31252 0.375023 0.390648 0.406259 0.414073 0.421883 0.429693 0.437504 0.445316 0.453129 0.460938 0.468749 0.476563 0.484374 0.5 0.515626 0.523437 0.531251 0.539062 0.546871 0.554684 0.562496 0.570307 0.578117 0.585927 0.593741 0.609352 0.624977 0.68748 0.749984 0.812488 0.874992 0.937496 1 1 1 1 projected
  arc A68 (571.4485, -220.4607) -> (574.9975, -211.031) centre (0, 0) ccw projected
  spline S65 degree 3 poles (574.9975, -211.031) (573.9773, -210.0839) (571.9369, -208.1897) (568.8113, -205.4194) (565.6369, -202.7057) (562.4085, -200.056) (559.121, -197.4804) (556.6226, -195.5908) (554.9207, -194.3813) (554.2662, -193.8033) (553.8116, -193.2747) (553.5193, -192.8417) (553.2554, -192.3902) (553.0594, -191.9051) (552.903, -191.4066) (552.8066, -190.8919) (552.7793, -190.3698) (552.7957, -189.8475) (552.8741, -189.3296) (553.0728, -188.6615) (553.3689, -187.8434) (553.632, -187.0142) (553.8811, -186.3632) (554.1341, -185.9046) (554.4391, -185.4802) (554.7786, -185.0826) (555.1683, -184.733) (555.5959, -184.4327) (556.0468, -184.1671) (556.531, -183.9696) (557.0265, -183.804) (557.7089, -183.6613) (558.58, -183.6013) (560.6665, -183.6777) (563.799, -183.6996) (567.975, -183.6575) (572.1493, -183.5207) (576.3198, -183.3002) (580.4859, -183.0051) (583.2578, -182.7445) (584.6438, -182.6141) knots 0 0 0 0 0.062504 0.125008 0.187512 0.250016 0.31252 0.375023 0.390648 0.406259 0.414073 0.421883 0.429693 0.437504 0.445316 0.453129 0.460938 0.468749 0.476563 0.484374 0.5 0.515626 0.523437 0.531251 0.539062 0.546871 0.554684 0.562496 0.570307 0.578117 0.585927 0.593741 0.609352 0.624977 0.68748 0.749984 0.812488 0.874992 0.937496 1 1 1 1 projected
  arc A69 (584.6438, -182.6141) -> (587.5685, -172.9726) centre (0, 0) ccw projected
  spline S66 degree 3 poles (587.5685, -172.9726) (586.4885, -172.0942) (584.3286, -170.3374) (581.0285, -167.7776) (577.6834, -165.2773) (574.2886, -162.8444) (570.8398, -160.4893) (568.223, -158.7672) (566.4457, -157.6715) (565.7548, -157.1376) (565.2666, -156.6399) (564.9466, -156.2269) (564.6538, -155.7937) (564.4264, -155.3224) (564.2377, -154.8352) (564.1079, -154.3279) (564.0466, -153.8087) (564.0288, -153.2864) (564.0731, -152.7645) (564.2277, -152.0848) (564.4696, -151.2492) (564.6779, -150.4045) (564.8839, -149.7386) (565.1064, -149.2645) (565.383, -148.8211) (565.6957, -148.402) (566.0618, -148.0277) (566.4688, -147.7001) (566.9013, -147.4056) (567.3716, -147.1769) (567.8552, -146.9792) (568.5268, -146.7922) (569.3921, -146.6753) (571.4792, -146.6151) (574.6064, -146.4321) (578.7707, -146.1169) (582.9271, -145.7074) (587.0743, -145.2146) (591.2121, -144.6477) (593.9611, -144.2063) (595.3355, -143.9856) knots 0 0 0 0 0.062504 0.125008 0.187512 0.250016 0.31252 0.375023 0.390648 0.406259 0.414073 0.421883 0.429693 0.437504 0.445316 0.453129 0.460938 0.468749 0.476563 0.484374 0.5 0.515626 0.523437 0.531251 0.539062 0.546871 0.554684 0.562496 0.570307 0.578117 0.585927 0.593741 0.609352 0.624977 0.68748 0.749984 0.812488 0.874992 0.937496 1 1 1 1 projected
  arc A70 (595.3355, -143.9856) -> (597.6234, -134.1734) centre (0, 0) ccw projected
  spline S67 degree 3 poles (597.6234, -134.1734) (596.4883, -133.3675) (594.2181, -131.7558) (590.7577, -129.4173) (587.2562, -127.1411) (583.7096, -124.9355) (580.114, -122.811) (577.3903, -121.2637) (575.5451, -120.2866) (574.8207, -119.7991) (574.3011, -119.3343) (573.9548, -118.9431) (573.6342, -118.53) (573.3765, -118.0746) (573.1564, -117.6007) (572.9936, -117.1031) (572.8985, -116.5889) (572.8465, -116.069) (572.8567, -115.5453) (572.9665, -114.857) (573.1532, -114.0073) (573.3059, -113.1508) (573.4678, -112.4728) (573.6589, -111.9851) (573.9058, -111.5246) (574.1905, -111.086) (574.5313, -110.6885) (574.916, -110.335) (575.3283, -110.0129) (575.7826, -109.7539) (576.2523, -109.525) (576.9102, -109.2945) (577.766, -109.1212) (579.8447, -108.9247) (582.9532, -108.5375) (587.088, -107.9507) (591.2087, -107.2701) (595.3148, -106.5072) (599.4067, -105.6709) (602.1209, -105.0506) (603.478, -104.7405) knots 0 0 0 0 0.062504 0.125008 0.187512 0.250016 0.31252 0.375023 0.390648 0.406259 0.414073 0.421883 0.429693 0.437504 0.445316 0.453129 0.460938 0.468749 0.476563 0.484374 0.5 0.515626 0.523437 0.531251 0.539062 0.546871 0.554684 0.562496 0.570307 0.578117 0.585927 0.593741 0.609352 0.624977 0.68748 0.749984 0.812488 0.874992 0.937496 1 1 1 1 projected
  arc A71 (603.478, -104.7405) -> (605.1192, -94.7997) centre (0, 0) ccw projected
  spline S68 degree 3 poles (605.1192, -94.7997) (603.9338, -94.0698) (601.5631, -92.61) (597.9571, -90.5028) (594.3142, -88.4605) (590.631, -86.4915) (586.9042, -84.6067) (584.0851, -83.2409) (582.1799, -82.3866) (581.4252, -81.9475) (580.8763, -81.5177) (580.5051, -81.15) (580.1582, -80.7587) (579.8713, -80.3212) (579.6206, -79.8627) (579.4257, -79.3768) (579.2971, -78.87) (579.2113, -78.3545) (579.1872, -77.8313) (579.2517, -77.1372) (579.3825, -76.2772) (579.4788, -75.4125) (579.5961, -74.7254) (579.7548, -74.2263) (579.9711, -73.7506) (580.2265, -73.2943) (580.5405, -72.8754) (580.9014, -72.4975) (581.2917, -72.1491) (581.7281, -71.8609) (582.1818, -71.6018) (582.8232, -71.3287) (583.6659, -71.0999) (585.7272, -70.7678) (588.8038, -70.1781) (592.8914, -69.3221) (596.9587, -68.3736) (601.0061, -67.3437) (605.0345, -66.2416) (607.7023, -65.4451) (609.0362, -65.0469) knots 0 0 0 0 0.062504 0.125008 0.187512 0.250016 0.31252 0.375023 0.390648 0.406259 0.414073 0.421883 0.429693 0.437504 0.445316 0.453129 0.460938 0.468749 0.476563 0.484374 0.5 0.515626 0.523437 0.531251 0.539062 0.546871 0.554684 0.562496 0.570307 0.578117 0.585927 0.593741 0.609352 0.624977 0.68748 0.749984 0.812488 0.874992 0.937496 1 1 1 1 projected
  arc A72 (609.0362, -65.0469) -> (610.0238, -55.02) centre (0, 0) ccw projected
  spline S69 degree 3 poles (610.0238, -55.02) (608.7932, -54.3692) (606.332, -53.0676) (602.596, -51.2007) (598.8274, -49.4011) (595.0232, -47.6772) (591.1811, -46.0402) (588.2787, -44.8617) (586.3218, -44.1338) (585.54, -43.745) (584.9641, -43.3521) (584.5697, -43.0094) (584.1979, -42.6417) (583.883, -42.2238) (583.6029, -41.7827) (583.3766, -41.3106) (583.2151, -40.8133) (583.0958, -40.3045) (583.0375, -39.784) (583.0565, -39.0872) (583.1308, -38.2204) (583.1703, -37.3513) (583.2424, -36.658) (583.3681, -36.1496) (583.5529, -35.6608) (583.7778, -35.1888) (584.0638, -34.7502) (584.3992, -34.3495) (584.7659, -33.9763) (585.1825, -33.6602) (585.6183, -33.3719) (586.2405, -33.0576) (587.0663, -32.7741) (589.1016, -32.3079) (592.133, -31.5183) (596.1558, -30.3968) (600.1524, -29.1842) (604.1238, -27.8919) (608.0715, -26.5286) (610.6815, -25.5594) (611.9865, -25.0748) knots 0 0 0 0 0.062504 0.125008 0.187512 0.250016 0.31252 0.375023 0.390648 0.406259 0.414073 0.421883 0.429693 0.437504 0.445316 0.453129 0.460938 0.468749 0.476563 0.484374 0.5 0.515626 0.523437 0.531251 0.539062 0.546871 0.554684 0.562496 0.570307 0.578117 0.585927 0.593741 0.609352 0.624977 0.68748 0.749984 0.812488 0.874992 0.937496 1 1 1 1 projected
  arc A73 (611.9865, -25.0748) -> (612.3162, -15.0048) centre (0, 0) ccw projected
  spline S70 degree 3 poles (612.3162, -15.0048) (611.0457, -14.4358) (608.5046, -13.298) (604.6545, -11.6794) (600.7762, -10.1301) (596.8674, -8.6588) (592.9265, -7.2766) (589.9533, -6.2904) (587.9529, -5.6921) (587.1474, -5.3552) (586.547, -5.0008) (586.131, -4.6846) (585.736, -4.342) (585.3945, -3.9456) (585.0861, -3.5238) (584.8294, -3.0675) (584.6357, -2.5818) (584.4834, -2.0819) (584.3912, -1.5663) (584.3646, -0.8698) (584.382, 0) (584.3646, 0.8698) (584.3912, 1.5663) (584.4834, 2.0819) (584.6357, 2.5818) (584.8294, 3.0675) (585.0861, 3.5238) (585.3945, 3.9456) (585.736, 4.342) (586.131, 4.6846) (586.547, 5.0008) (587.1474, 5.3552) (587.9529, 5.6921) (589.9533, 6.2904) (592.9265, 7.2766) (596.8674, 8.6588) (600.7762, 10.1301) (604.6545, 11.6794) (608.5046, 13.298) (611.0457, 14.4358) (612.3162, 15.0048) knots 0 0 0 0 0.062504 0.125008 0.187512 0.250016 0.31252 0.375023 0.390648 0.406259 0.414073 0.421883 0.429693 0.437504 0.445316 0.453129 0.460938 0.468749 0.476563 0.484374 0.5 0.515626 0.523437 0.531251 0.539062 0.546871 0.554684 0.562496 0.570307 0.578117 0.585927 0.593741 0.609352 0.624977 0.68748 0.749984 0.812488 0.874992 0.937496 1 1 1 1 projected
  arc A74 (612.3162, 15.0048) -> (611.9865, 25.0748) centre (0, 0) ccw projected